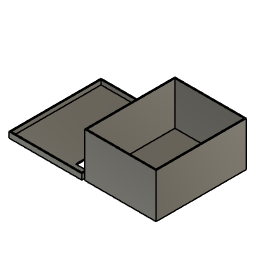
PCB-Case (Autodesk Fusion 360 design; units mm, degrees)
part number: 2025-06-10-07-03-33-286
Autodesk Fusion 360 part; units mm, degrees
box "BoxPrimitive1" add length 81.5 width 64.5 height 5 placed x (0, 1, 0) y (-1, 0, 0) z (0, 0, 1) at (0, 0, 0) makes body 1
extrude "Extrude1" add 1 faces at (-21.5, 27.1667, 5) along direction (0, 0, 1) blind 35 on bodies 1 bodies 1
shell "Shell1" thickness 1 removed faces 1 at (-21.5, 27.1667, 40) on bodies 1
box "BoxPrimitive2" add length 81.5 width 64.5 height 5 placed x (0, -1, 0) y (1, 0, 0) z (0, 0, 1) at (-64.5, 81.5, 40) separate body makes body 2
scale "Scale1" factor 1.02 about (0, 0, 45) bodies 2
move_body "Move1" bodies 2 to x (1, 0, 0) y (0, 1, 0) z (0, 0, 1) at (-67.4054, -1.0007, -40)
shell "Shell2" thickness 1 removed faces 1 at (-89.3354, 54.4193, 5) on bodies 2
scale "Scale2" factor 1.02 about (-1, 1, 1) bodies 1
scale "Scale3" factor 1.02 about (-68.4054, -0.0007, 0.9) bodies 2
hole "Hole1" at (-62.2928, 4.489, 1) direction (0, 0, -1) diameter 2.5 depth 10 tip angle 118 bodies 1
hole "Hole2" at (-36.6483, 4.4332, 1) direction (0, 0, -1) diameter 2.5 depth 1.02 tip angle 118 bodies 1
box "BoxPrimitive4" cut length 66 width 10 height -1.02 placed x (0, -1, 0) y (1, 0, 0) z (0, 0, 1) at (-82, 74, 0.9) bodies 2
sketch "Sketch4" plane through (0, 0, 0) normal (0, 0, 1) x (1, 0, 0)
  line L0 (23.331, -0.5035) -> (102.831, -0.5035)
  line L1 (102.831, -0.5035) -> (102.831, 61.9965)
  line L2 (102.831, 61.9965) -> (23.331, 61.9965)
  line L3 (23.331, 61.9965) -> (23.331, -0.5035)
  dimension "d17" = 79.5
  dimension "d18" = 62.5
  constraint horizontal L0
  constraint vertical L1
  constraint horizontal L2
  constraint vertical L3
  measures "d17" distance of L0.start L0.end
  measures "d18" distance of L0.start L2.end
